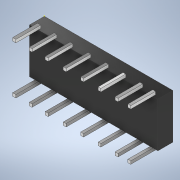
# Autodesk Inventor part: hbridge
Saved by Autodesk Inventor 2021 (Build 250183000, 183)
## iProperties
Created: 2021-07-15
Part Number: hbridge
Material: Generic
Document SubType Name: Modeling
Designer: HP
Density: 1 g/cm^3
Appearance: Default
Author: HP
Autodesk Inventor part; units mm, degrees
ref_plane "YZ Plane" through (0, 0, 0) normal (1, 0, 0) x (0, 1, 0)
ref_plane "XZ Plane" through (0, 0, 0) normal (0, 1, 0) x (-1, 0, 0)
ref_plane "XY Plane" through (0, 0, 0) normal (0, 0, 1) x (1, 0, 0)
sketch "Sketch1" plane through (0, 0, 0) normal (0, 0, 1) x (1, 0, 0)
  line L0 (0, 0) -> (43, 0)
  line L1 (43, 0) -> (43, 15)
  line L2 (43, 15) -> (0, 15)
  line L3 (0, 15) -> (0, 0)
  dimension "d0" = 43
  dimension "d1" = 15
  constraints: 8 end point, 2 parallel, 1 horizontal, 1 perpendicular
  measures "d0" distance of L2.end L1.end
  measures "d1" distance of L1.end L0.end
extrude "Extrusion1" add sketch "Sketch1" along normal blind 5
sketch "Sketch2" plane through (0, 15, 0) normal (0, 1, 0) x (1, 0, 0)
  point P0 (0, 0)
sketch "Sketch3" plane through (0, 15, 0) normal (0, 1, 0) x (1, 0, 0)
  line L0 (1.8425, -12.4637) -> (1.8425, -4.1304)
  line L1 (1.8425, -4.1304) -> (2.9382, -4.1304)
  line L2 (2.9382, -4.1304) -> (2.9382, -12.4637)
  line L3 (2.9382, -12.4637) -> (1.8425, -12.4637)
  line L4 (1.8425, -12.4637) -> (1.8425, -4.1304)
  line L5 (7.4078, -4.1304) -> (8.3192, -4.1304)
  line L6 (8.3192, -4.1304) -> (8.3192, -12.4637)
  line L7 (8.3192, -12.4637) -> (7.4078, -12.4637)
  line L8 (7.4078, -12.4637) -> (7.4078, -4.1304)
  line L9 (12.7537, -4.1304) -> (13.7002, -4.1304)
  line L10 (13.7002, -4.1304) -> (13.7002, -12.4637)
  line L11 (13.7002, -12.4637) -> (12.7537, -12.4637)
  line L12 (12.7537, -12.4637) -> (12.7537, -4.1304)
  line L13 (18.7833, -4.1304) -> (19.7298, -4.1304)
  line L14 (19.7298, -4.1304) -> (19.7298, -12.4637)
  line L15 (19.7298, -12.4637) -> (18.7833, -12.4637)
  line L16 (18.7833, -12.4637) -> (18.7833, -4.1304)
  line L17 (24.6292, -4.1304) -> (25.5788, -4.1304)
  line L18 (25.5788, -4.1304) -> (25.5788, -12.4637)
  line L19 (25.5788, -12.4637) -> (24.6292, -12.4637)
  line L20 (24.6292, -12.4637) -> (24.6292, -4.1304)
  line L21 (30.4626, -4.1304) -> (31.367, -4.1304)
  line L22 (31.367, -4.1304) -> (31.367, -12.4637)
  line L23 (31.367, -12.4637) -> (30.4626, -12.4637)
  line L24 (30.4626, -12.4637) -> (30.4626, -4.1304)
  line L25 (36.1151, -4.1304) -> (37.11, -4.1304)
  line L26 (37.11, -4.1304) -> (37.11, -12.4637)
  line L27 (37.11, -12.4637) -> (36.1151, -12.4637)
  line L28 (36.1151, -12.4637) -> (36.1151, -4.1304)
  line L29 (40.4111, -4.1304) -> (41.3607, -4.1304)
  line L30 (41.3607, -4.1304) -> (41.3607, -12.4637)
  line L31 (41.3607, -12.4637) -> (40.4111, -12.4637)
  line L32 (40.4111, -12.4637) -> (40.4111, -4.1304)
  line L33 (1.8425, -4.1304) -> (2.9382, -4.1304)
  line L34 (7.4078, -4.1304) -> (8.3192, -4.1304)
  line L35 (12.7537, -4.1304) -> (13.7002, -4.1304)
  line L36 (18.7833, -4.1304) -> (19.7298, -4.1304)
  line L37 (24.6292, -4.1304) -> (25.5788, -4.1304)
  line L38 (30.4626, -4.1304) -> (31.367, -4.1304)
  line L39 (36.1151, -4.1304) -> (37.11, -4.1304)
  line L40 (40.4111, -4.1304) -> (41.3607, -4.1304)
  line L41 (41.3607, -12.4637) -> (40.4111, -12.4637)
  line L42 (37.11, -12.4637) -> (36.1151, -12.4637)
  line L43 (31.367, -12.4637) -> (30.4626, -12.4637)
  line L44 (25.5788, -12.4637) -> (24.6292, -12.4637)
  line L45 (19.7298, -12.4637) -> (18.7833, -12.4637)
  line L46 (13.7002, -12.4637) -> (12.7537, -12.4637)
  line L47 (8.3192, -12.4637) -> (7.4078, -12.4637)
  line L48 (2.9382, -12.4637) -> (1.8425, -12.4637)
  point P0 (0, 0)
  constraints: 98 end point, 80 parallel, 16 horizontal, 8 perpendicular
extrude "Extrusion2" add sketch "Sketch3" along normal blind 1
sketch "Sketch4" plane through (0, 0, 0) normal (0, -1, 0) x (1, 0, 0)
  line L0 (41.3607, 4.1304) -> (40.4111, 4.1304) projected
  line L1 (40.4111, 4.1304) -> (40.4111, 12.4637) projected
  line L2 (41.3607, 4.1304) -> (40.4111, 4.1304)
  line L3 (40.4111, 4.1304) -> (40.4111, 12.4637)
  line L4 (40.4111, 12.4637) -> (41.3607, 12.4637)
  line L5 (41.3607, 12.4637) -> (41.3607, 4.1304)
  line L6 (36.1151, 4.1304) -> (37.11, 4.1304) projected
  line L7 (36.1151, 5) -> (36.1151, 12.4637) projected
  line L8 (37.11, 4.1304) -> (36.1151, 4.1304)
  line L9 (36.1151, 4.1304) -> (36.1151, 12.4637)
  line L10 (36.1151, 12.4637) -> (37.11, 12.4637)
  line L11 (37.11, 12.4637) -> (37.11, 4.1304)
  line L12 (30.4626, 4.1304) -> (30.4626, 12.4637) projected
  line L13 (31.367, 4.1304) -> (30.4626, 4.1304)
  line L14 (30.4626, 4.1304) -> (30.4626, 12.4637)
  line L15 (30.4626, 12.4637) -> (31.367, 12.4637)
  line L16 (31.367, 12.4637) -> (31.367, 4.1304)
  line L17 (25.5788, 4.1304) -> (24.6292, 4.1304) projected
  line L18 (24.6292, 4.1304) -> (24.6292, 12.4637) projected
  line L19 (25.5788, 4.1304) -> (24.6292, 4.1304)
  line L20 (24.6292, 4.1304) -> (24.6292, 12.4637)
  line L21 (24.6292, 12.4637) -> (25.5788, 12.4637)
  line L22 (25.5788, 12.4637) -> (25.5788, 4.1304)
  line L23 (19.7298, 12.4637) -> (19.7298, 4.1304) projected
  line L24 (18.7833, 4.1304) -> (18.7833, 12.4637) projected
  line L25 (19.7298, 4.1304) -> (18.7833, 4.1304)
  line L26 (18.7833, 4.1304) -> (18.7833, 12.4637)
  line L27 (18.7833, 12.4637) -> (19.7298, 12.4637)
  line L28 (19.7298, 12.4637) -> (19.7298, 4.1304)
  line L29 (13.7002, 4.1304) -> (13.7002, 5) projected
  line L30 (12.7537, 4.1304) -> (12.7537, 12.4637) projected
  line L31 (13.7002, 4.1304) -> (12.7537, 4.1304)
  line L32 (12.7537, 4.1304) -> (12.7537, 12.4637)
  line L33 (12.7537, 12.4637) -> (13.7002, 12.4637)
  line L34 (13.7002, 12.4637) -> (13.7002, 4.1304)
  line L35 (8.3192, 4.1304) -> (8.3192, 5) projected
  line L36 (7.4078, 4.1304) -> (7.4078, 12.4637) projected
  line L37 (8.3192, 4.1304) -> (7.4078, 4.1304)
  line L38 (7.4078, 4.1304) -> (7.4078, 12.4637)
  line L39 (7.4078, 12.4637) -> (8.3192, 12.4637)
  line L40 (8.3192, 12.4637) -> (8.3192, 4.1304)
  line L41 (2.9382, 4.1304) -> (1.8425, 4.1304) projected
  line L42 (1.8425, 4.1304) -> (1.8425, 12.4637) projected
  line L43 (2.9382, 4.1304) -> (1.8425, 4.1304)
  line L44 (1.8425, 4.1304) -> (1.8425, 12.4637)
  line L45 (1.8425, 12.4637) -> (2.9382, 12.4637)
  line L46 (2.9382, 12.4637) -> (2.9382, 4.1304)
  point P0 (0, 0)
  constraints: 64 end point, 16 parallel, 8 horizontal, 8 perpendicular
extrude "Extrusion3" add sketch "Sketch4" along normal blind 1
body "Solid1"
